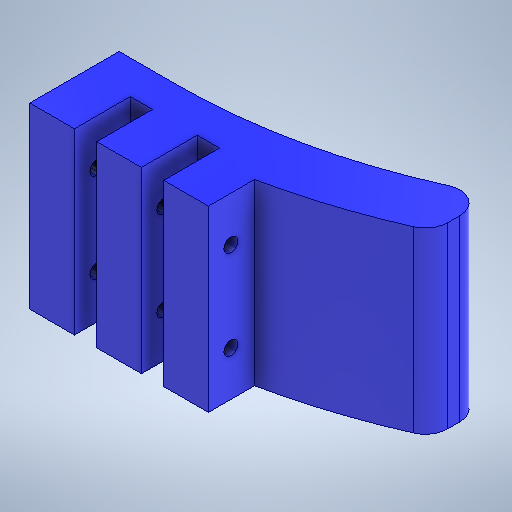
# Autodesk Inventor part: hand2_14
Saved by Autodesk Inventor 2025.1 (Build 291241000, 241)
## iProperties
Created: 2025-02-05
Part Number: hand2_14
Material: ABS プラスチック
Document SubType Name: Modeling
Designer: ryogo
Density: 1.06 g/cm^3
Appearance: 青 - 壁塗料 - 光沢
Author: ryogo
Autodesk Inventor part; units mm, degrees
ref_plane "YZ Plane" through (0, 0, 0) normal (1, 0, 0) x (0, 1, 0)
ref_plane "XZ Plane" through (0, 0, 0) normal (0, 1, 0) x (-1, 0, 0)
ref_plane "XY Plane" through (0, 0, 0) normal (0, 0, 1) x (1, 0, 0)
sketch "スケッチ3" plane through (0, 0, 0) normal (0, 1, 0) x (-1, 0, 0)
  line L0 (0, 0) -> (25, 0)
  line L1 (25, 0) -> (25, -12.5)
  line L2 (25, -12.5) -> (0, -12.5)
  line L3 (0, -12.5) -> (0, 0)
  line L4 (15, 0) -> (10, 0)
  line L5 (10, 0) -> (10, -12.5)
  line L6 (10, -12.5) -> (15, -12.5)
  line L7 (15, -12.5) -> (15, 0)
  dimension "d112" = 25
  dimension "d113" = 12.5
  dimension "d114" = 5
  dimension "d115" = 10
  constraints: 16 end point, 4 parallel, 2 horizontal, 2 perpendicular, 2 point on line
  measures "d112" distance of L1.end L2.end
  measures "d113" distance between parallel lines of L0 L2
  measures "d114" distance of L6.end L5.end
  measures "d115" distance between parallel lines of L7 L1
extrude "押し出し1" add sketch "スケッチ3" along normal blind 40 contours L0 L5 L2 L3 | L0 L1 L2 L7
sketch "スケッチ4" plane through (0, 0, 0) normal (1, 0, 0) x (0, 0, -1)
  line L0 (12.5, 0) -> (0, 0) projected
  line L1 (5, 0) -> (5, 40)
  line L2 (0, 40) -> (12.5, 40) projected
  line L3 (12.5, 0) -> (12.5, 40) projected
  line L4 (0, 0) -> (0, 40) projected
  line L5 (0, 20) -> (12.5, 20)
  point P0 (5, 30)
  point P1 (5, 10)
  dimension "d118" = 7.5
  dimension "d119" = 20
  dimension "d120" = 20
  constraints: 4 end point, 4 point on line, 2 midpoint, 1 vertical
  measures "d118" distance between parallel lines of L3 L1
  measures "d119" diameter of point (5, 30) L5
  measures "d120" diameter of point (5, 10) L5
hole "穴1" at (0, 30, -5) at (0, 10, -5) direction (-1, 0, 0) diameter 3.1 end through all
sketch "スケッチ5" plane through (0, 0, 0) normal (0, -1, 0) x (1, 0, 0)
  line L0 (0, -12.5) -> (-10, -12.5) projected
  line L1 (0, -12.5) -> (-25, -12.5)
  line L2 (-25, -12.5) -> (-25, -17.5)
  line L3 (-25, -17.5) -> (0, -17.5)
  line L4 (0, -17.5) -> (0, -12.5)
  point P0 (0, 0)
  dimension "d128" = 5
  constraints: 8 end point, 2 parallel, 1 horizontal, 1 perpendicular
  measures "d128" distance of L2.end L1.end
extrude "押し出し2" add sketch "スケッチ5" against normal blind 40
sketch "スケッチ6" plane through (0, 0, 0) normal (0, -1, 0) x (1, 0, 0)
  line L0 (-15, -12.5) -> (-10, -12.5) projected
  line L1 (-12.5, -12.5) -> (-12.5, -232.0211)
  circle A0 centre (-12.5, -142.5) radius 122.5
  line L2 (-25, -17.5) -> (0, -17.5) projected
  circle A1 centre (-12.5, -142.5) radius 135
  line L3 (0, 0) -> (0, -17.5) projected
  line L4 (0, -17.5) -> (5, -17.5)
  line L5 (5, -17.5) -> (5, -12.5)
  line L6 (5, -12.5) -> (0, -12.5)
  line L7 (0, -12.5) -> (0, -17.5)
  line L8 (5, -17.5) -> (15, -17.5)
  line L9 (15, -17.5) -> (15, 0)
  line L10 (15, 0) -> (5, 0)
  line L11 (5, 0) -> (5, -17.5)
  line L12 (45, -20.3577) -> (45, -34.3335)
  line L13 (-12.5, -20) -> (-25, -20)
  line L14 (-25, 0) -> (-25, -17.5) projected
  line L15 (-25, -20) -> (-25, -17.5)
  point P0 (0, -12.5)
  point P1 (-12.5, -17.5)
  point P2 (15, -10.3306)
  point P3 (0, -8.0799)
  point P4 (5, -8.6391)
  dimension "d132" = 270
  dimension "d131" = 245
  dimension "d133" = 5
  dimension "d134" = 5
  dimension "d135" = 10
  dimension "d136" = 17.5
  dimension "d139" = 30
  dimension "d144" = 125
  constraints: 24 end point, 4 parallel, 3 horizontal, 3 perpendicular, 2 point on circle, 2 point on line, 2 vertical, 1 centre point, 1 coincident, 1 midpoint, 3 other
  measures "d131" diameter of A0
  measures "d133" distance between parallel lines of L3 L5
  measures "d134" distance between parallel lines of L4 L6
  measures "d135" distance of L10.end L9.end
  measures "d136" distance between parallel lines of L10 L8
  measures "d139" distance between parallel lines of L9 L12
  measures "d144" distance from line of L2 A0.centre
extrude "押し出し3" add sketch "スケッチ6" against normal blind 40 contours L3 L6 L5 L4 | L5 L11 A1 L9 L8 | A1 L11 L10 L9
extrude "押し出し4" add sketch "スケッチ6" against normal blind 40 contours L2 L4 L8 L9 A1 L12 A0 L1 | L1 L13 L15 L2
sketch "スケッチ7" plane through (15, 0, 0) normal (1, 0, 0) x (0, 0, -1)
  circle A0 centre (5, 30) radius 1.55 projected
  circle A1 centre (5, 10) radius 1.55 projected
  point P0 (0, 0)
extrude "押し出し5" cut sketch "スケッチ7" against normal blind 40
fillet "フィレット1" radius 5 1 edges at (45, 20, -34.3335)
fillet "フィレット2" radius 5 1 edges at (45, 20, -20.3577)
